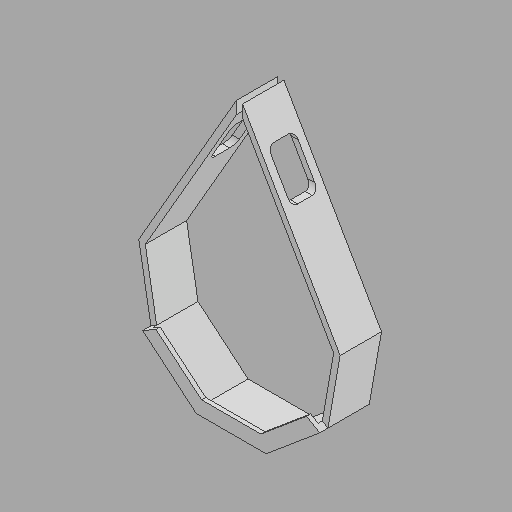
# Autodesk Inventor part: HARNESS
Saved by Autodesk Inventor 2025.2 (Build 292293000, 293)
## iProperties
Created: 2026-06-28
Part Number: HARNESS
Material: Generic
Document SubType Name: Modeling
Designer: Ben
Density: 1 g/cm^3
Appearance: Default
Author: Ben
Autodesk Inventor part; units mm, degrees
ref_plane "YZ Plane" through (0, 0, 0) normal (1, 0, 0) x (0, 1, 0)
ref_plane "XZ Plane" through (0, 0, 0) normal (0, 1, 0) x (-1, 0, 0)
ref_plane "XY Plane" through (0, 0, 0) normal (0, 0, 1) x (1, 0, 0)
sketch "Sketch1" plane through (0, 0, 0) normal (0, 0, 1) x (1, 0, 0)
  line L0 (29.7558, 35.4616) -> (45.5886, 8.0385)
  line L1 (45.5886, 8.0385) -> (40.0899, -23.1459)
  line L2 (40.0899, -23.1459) -> (15.8328, -43.5001)
  line L3 (15.8328, -43.5001) -> (-15.8328, -43.5001)
  line L4 (-15.8328, -43.5001) -> (-40.0899, -23.1459)
  line L5 (-40.0899, -23.1459) -> (-45.5886, 8.0385)
  line L6 (-45.5886, 8.0385) -> (-29.7558, 35.4616)
  line L7 (-29.7558, 35.4616) -> (0, 46.2919)
  line L8 (0, 46.2919) -> (29.7558, 35.4616)
  line L9 (-29.7558, 35.4616) -> (0, 87.0003)
  line L10 (0, 87.0003) -> (29.7558, 35.4616)
  line L11 (0, 93.0003) -> (-48.7326, 8.5929)
  line L12 (-48.7326, 8.5929) -> (-42.8548, -24.7422)
  line L13 (-42.8548, -24.7422) -> (-16.9247, -46.5001)
  line L14 (-16.9247, -46.5001) -> (16.9247, -46.5001)
  line L15 (16.9247, -46.5001) -> (42.8548, -24.7422)
  line L16 (42.8548, -24.7422) -> (48.7326, 8.5929)
  line L17 (48.7326, 8.5929) -> (0, 93.0003)
  line L18 (0, -74.4002) -> (0, 120.9003) projected
  point P0 (0, 0)
  point P1 (0, 0)
  dimension "d0" = 89.792
  dimension "d1" = 3
  dimension "d2" = 3
  dimension "d3" = 3
  dimension "d4" = 3
  constraints: 36 end point, 3 parallel, 2 collinear, 1 coincident, 1 horizontal, 1 vertical alignment, 22 other
  measures "d0" distance from line of L3 L7.end
  measures "d1" distance between parallel lines of L9 L11
  measures "d2" distance between parallel lines of L12 L5
  measures "d3" distance between parallel lines of L13 L4
  measures "d4" distance between parallel lines of L14 L3
extrude "Extrusion1" add sketch "Sketch1" along normal mid plane 20 contours L10 L18 L17 L16 L15 L14 L3 L2 L1 L0 | L9 L6 L5 L4 L3 L18 L14 L13 L12 L11
sketch "Sketch2" plane through (0, 0, 10) normal (0, 0, 1) x (1, 0, 0)
  line L0 (-1.5, 90.4022) -> (-1.5, 84.4022)
  line L1 (0, 87.0003) -> (-45.5886, 8.0385) projected
  line L2 (45.5886, 8.0385) -> (0, 87.0003) projected
  line L3 (1.5, 84.4022) -> (1.5, 90.4022)
  line L4 (48.7326, 8.5929) -> (0, 93.0003) projected
  line L5 (16.9247, -46.5001) -> (42.8548, -24.7422) projected
  line L6 (42.8548, -24.7422) -> (48.7326, 8.5929) projected
  line L7 (48.7326, 8.5929) -> (0, 93.0003) projected
  line L8 (0, 93.0003) -> (-48.7326, 8.5929) projected
  line L9 (-48.7326, 8.5929) -> (-42.8548, -24.7422) projected
  line L10 (-42.8548, -24.7422) -> (-16.9247, -46.5001) projected
  line L11 (-16.9247, -46.5001) -> (16.9247, -46.5001) projected
  line L12 (15.8328, -43.5001) -> (-15.8328, -43.5001) projected
  line L13 (-15.8328, -43.5001) -> (-40.0899, -23.1459) projected
  line L14 (-40.0899, -23.1459) -> (-45.5886, 8.0385) projected
  line L15 (-45.5886, 8.0385) -> (0, 87.0003) projected
  line L16 (0, 87.0003) -> (45.5886, 8.0385) projected
  line L17 (45.5886, 8.0385) -> (40.0899, -23.1459) projected
  line L18 (40.0899, -23.1459) -> (15.8328, -43.5001) projected
  line L19 (0, -74.4002) -> (0, 120.9003) projected
  point P0 (0, 0)
  dimension "d7" = 3
  constraints: 4 end point, 4 point on line, 1 parallel, 1 vertical, 1 other
  measures "d7" distance between parallel lines of L3 L0
extrude "Extrusion2" cut sketch "Sketch2" against normal through all contours L8 L19 L1 L0 | L4 L3 L2 L19
sketch "Sketch3" plane through (0, 0, 0) normal (1, 0, 0) x (0, 1, 0)
  line L0 (90.4022, -10) -> (90.4022, 10) projected
  line L1 (8.5929, 10) -> (90.4022, 10) projected
  line L2 (8.5929, -10) -> (8.5929, 10) projected
  line L3 (90.4022, -10) -> (8.5929, -10) projected
  line L4 (55.4022, 6.5) -> (75.4022, 6.5)
  line L5 (75.4022, 6.5) -> (75.4022, -6.5)
  line L6 (75.4022, -6.5) -> (55.4022, -6.5)
  line L7 (55.4022, -6.5) -> (55.4022, 6.5)
  line L8 (55.4022, 6.5) -> (75.4022, -6.5) construction
  line L9 (75.4022, 6.5) -> (55.4022, -6.5) construction
  point P0 (0, 0)
  point P1 (65.4022, 0)
  point P2 (90.4022, 0)
  dimension "d10" = 13
  dimension "d11" = 15
  dimension "d12" = 20
  constraints: 12 end point, 3 midpoint, 2 parallel, 1 horizontal, 1 horizontal alignment, 1 perpendicular
  measures "d10" distance between parallel lines of L6 L4
  measures "d11" distance between parallel lines of L5 L0
  measures "d12" distance of L5.end L6.end
extrude "Extrusion3" cut sketch "Sketch3" along normal through all both and the other way through all contours L4 L5 L6 L7
fillet "Fillet1" radius 3 8 edges at (8.4282, 75.4022, 6.5) (19.9752, 55.4022, 6.5) (19.9752, 55.4022, -6.5) (8.4282, 75.4022, -6.5) (-8.4282, 75.4022, -6.5) (-8.4282, 75.4022, 6.5) (-19.9752, 55.4022, 6.5) (-19.9752, 55.4022, -6.5)
sketch "Sketch5" plane through (0, 0, 10) normal (0, 0, 1) x (1, 0, 0)
  line L0 (1.5, 90.4022) -> (1.5, 84.4022) projected
  line L1 (1.5, 84.4022) -> (45.5886, 8.0385) projected
  line L2 (45.5886, 8.0385) -> (40.0899, -23.1459) projected
  line L3 (40.0899, -23.1459) -> (15.8328, -43.5001) projected
  line L4 (15.8328, -43.5001) -> (-15.8328, -43.5001) projected
  line L5 (-15.8328, -43.5001) -> (-40.0899, -23.1459) projected
  line L6 (-40.0899, -23.1459) -> (-45.5886, 8.0385) projected
  line L7 (-45.5886, 8.0385) -> (-1.5, 84.4022) projected
  line L8 (-1.5, 84.4022) -> (-1.5, 90.4022) projected
  line L9 (-1.5, 90.4022) -> (-48.7326, 8.5929) projected
  line L10 (-48.7326, 8.5929) -> (-42.8548, -24.7422) projected
  line L11 (-42.8548, -24.7422) -> (-16.9247, -46.5001) projected
  line L12 (-16.9247, -46.5001) -> (16.9247, -46.5001) projected
  line L13 (16.9247, -46.5001) -> (42.8548, -24.7422) projected
  line L14 (42.8548, -24.7422) -> (48.7326, 8.5929) projected
  line L15 (48.7326, 8.5929) -> (1.5, 90.4022) projected
  line L16 (-40.0899, -23.1459) -> (-42.8548, -24.7422)
  line L17 (40.0899, -23.1459) -> (45.5886, 8.0385) projected
  line L18 (40.0899, -23.1459) -> (42.8548, -24.7422)
  point P0 (0, 0)
  constraints: 4 end point
extrude "Extrusion5" add sketch "Sketch5" along normal blind 2 contours L13 L12 L11 L16 L5 L4 L3 L18
sketch "Sketch6" plane through (0, 0, 12) normal (0, 0, 1) x (1, 0, 0)
  line L0 (15.8328, -43.5001) -> (-15.8328, -43.5001) projected
  line L1 (-15.8328, -43.5001) -> (-40.0899, -23.1459) projected
  line L2 (-40.0899, -23.1459) -> (-42.8548, -24.7422) projected
  line L3 (-42.8548, -24.7422) -> (-16.9247, -46.5001) projected
  line L4 (-16.9247, -46.5001) -> (16.9247, -46.5001) projected
  line L5 (16.9247, -46.5001) -> (42.8548, -24.7422) projected
  line L6 (42.8548, -24.7422) -> (40.0899, -23.1459) projected
  line L7 (40.0899, -23.1459) -> (15.8328, -43.5001) projected
  line L8 (-42.8548, -24.7422) -> (-36.4035, -21.0176)
  line L9 (-36.4035, -21.0176) -> (-14.3769, -39.5001)
  line L10 (-14.3769, -39.5001) -> (14.3769, -39.5001)
  line L11 (14.3769, -39.5001) -> (36.4035, -21.0176)
  line L12 (36.4035, -21.0176) -> (42.8548, -24.7422)
  line L13 (-40.0899, -23.1459) -> (-42.8548, -24.7422) projected
  line L14 (0, -73.8806) -> (0, 117.7826) projected
  point P0 (0, 0)
  dimension "d21" = 4
  dimension "d22" = 4
  constraints: 10 end point, 2 collinear, 1 horizontal, 1 other
  measures "d21" distance between parallel lines of L1 L9
  measures "d22" distance between parallel lines of L0 L10
extrude "Extrusion6" add sketch "Sketch6" along normal blind 2
body "Solid1"
